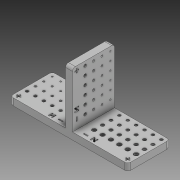
# Autodesk Inventor part: Drill Bushings Test Print
Saved by Autodesk Inventor 2022 (Build 260153000, 153)
## iProperties
Created: 2022-01-18
Part Number: Drill Bushings Test Print
Material: ABS Plastic
Document SubType Name: Modeling
Density: 1.06 g/cm^3
Appearance: Smooth - Medium Gray
Autodesk Inventor part; units mm, degrees
ref_plane "YZ Plane" through (0, 0, 0) normal (1, 0, 0) x (0, 1, 0)
ref_plane "XZ Plane" through (0, 0, 0) normal (0, 1, 0) x (-1, 0, 0)
ref_plane "XY Plane" through (0, 0, 0) normal (0, 0, 1) x (1, 0, 0)
sketch "Sketch1" plane through (0, 0, 0) normal (0, 1, 0) x (-1, 0, 0)
  line L0 (4.7625, 77.3906) -> (-4.7625, 77.3906)
  line L1 (-4.7625, 77.3906) -> (-4.7625, 75.0094)
  line L2 (-4.7625, 75.0094) -> (4.7625, 75.0094)
  line L3 (4.7625, 75.0094) -> (4.7625, 77.3906)
  line L4 (4.7625, 77.3906) -> (-4.7625, 75.0094) construction
  line L5 (-4.7625, 77.3906) -> (4.7625, 75.0094) construction
  line L6 (-90.4875, 77.3906) -> (-100.0125, 77.3906)
  line L7 (-100.0125, 77.3906) -> (-100.0125, 75.0094)
  line L8 (-100.0125, 75.0094) -> (-90.4875, 75.0094)
  line L9 (-90.4875, 75.0094) -> (-90.4875, 77.3906)
  line L10 (-90.4875, 77.3906) -> (-100.0125, 75.0094) construction
  line L11 (-100.0125, 77.3906) -> (-90.4875, 75.0094) construction
  line L12 (-96.4406, 71.4375) -> (-94.0594, 71.4375)
  line L13 (-94.0594, 71.4375) -> (-94.0594, 80.9625)
  line L14 (-94.0594, 80.9625) -> (-96.4406, 80.9625)
  line L15 (-96.4406, 80.9625) -> (-96.4406, 71.4375)
  line L16 (-96.4406, 71.4375) -> (-94.0594, 80.9625) construction
  line L17 (-94.0594, 71.4375) -> (-96.4406, 80.9625) construction
  line L18 (-14.2875, 80.9625) -> (-14.2875, 71.4375)
  line L19 (-14.2875, 71.4375) -> (-16.6687, 71.4375)
  line L20 (-16.6687, 71.4375) -> (-21.4312, 77.2177)
  line L21 (-21.4312, 77.2177) -> (-21.4312, 71.4375)
  line L22 (-21.4312, 71.4375) -> (-23.8125, 71.4375)
  line L23 (-23.8125, 71.4375) -> (-23.8125, 80.9625)
  line L24 (-23.8125, 80.9625) -> (-21.4312, 80.9625)
  line L25 (-21.4312, 80.9625) -> (-16.6687, 75.1823)
  line L26 (-16.6687, 75.1823) -> (-16.6687, 80.9625)
  line L27 (-16.6687, 80.9625) -> (-14.2875, 80.9625)
  line L28 (-19.05, 78.0724) -> (-19.05, 74.3276) construction
  line L29 (28.575, -9.525) -> (-104.775, -9.525)
  line L30 (-104.775, -9.525) -> (-104.775, 85.725)
  line L31 (-104.775, 85.725) -> (28.575, 85.725)
  line L32 (28.575, 85.725) -> (28.575, -9.525)
  line L33 (28.575, -9.525) -> (-104.775, 85.725) construction
  line L34 (-104.775, -9.525) -> (28.575, 85.725) construction
  point P0 (0, 76.2)
  point P1 (-95.25, 76.2)
  point P2 (-95.25, 76.2)
  point P3 (0, 76.2)
  point P4 (-95.25, 76.2)
  point P5 (0, 76.2)
  point P6 (-95.25, 76.2)
  point P7 (-96.4406, 77.3906)
  point P8 (-94.0594, 77.3906)
  point P9 (-94.0594, 75.0094)
  point P10 (-96.4406, 75.0094)
  point P11 (0, 0)
  point P12 (-19.05, 76.2)
  point P13 (-95.25, 76.2)
  point P14 (-19.05, 0)
  point P15 (-38.1, 0)
  point P16 (-57.15, 0)
  point P17 (-76.2, 0)
  point P18 (-38.1, 38.1)
  point P19 (-95.25, 0)
  point P20 (0, 19.05)
  point P21 (-19.05, 19.05)
  point P22 (-57.15, 19.05)
  point P23 (-38.1, 19.05)
  point P24 (-95.25, 19.05)
  point P25 (-76.2, 19.05)
  point P26 (0, 38.1)
  point P27 (-19.05, 38.1)
  point P28 (-57.15, 38.1)
  point P29 (-38.1, 38.1)
  point P30 (-95.25, 38.1)
  point P31 (-76.2, 38.1)
  point P32 (0, 57.15)
  point P33 (-19.05, 57.15)
  point P34 (-57.15, 57.15)
  point P35 (-38.1, 57.15)
  point P36 (-95.25, 57.15)
  point P37 (-76.2, 57.15)
  point P38 (28.575, 38.1)
  dimension "d137" = 25.4
  dimension "d33" = 9.525
  dimension "d34" = 2.3813
  dimension "d61" = 9.525
  dimension "d62" = 9.525
  dimension "d64" = 2.3813
  dimension "d67" = 133.35
  dimension "d81" = 19.05
  dimension "d123" = 0
  dimension "d134" = 19.05
  dimension "d139" = 19.05
  dimension "d140" = 9.525
  constraints: 71 end point, 17 midpoint, 11 parallel, 7 equal length, 7 perpendicular, 6 point on line, 5 horizontal, 4 vertical alignment, 3 horizontal alignment, 2 vertical, 23 other
  measures "d33" distance of L1.end L2.end
  measures "d34" distance of L2.end L0.start
  measures "d61" distance between parallel lines of L23 L18
  measures "d62" distance between parallel lines of L24 L22
  measures "d64" distance between parallel lines of L25 L20
  measures "d67" distance of L29.start L29.end
  measures "d81" distance of point (0, 0) point (-19.05, 0)
  measures "d123" horizontal distance of point (-38.1, 38.1) point (-38.1, 0)
  measures "d134" distance of point (0, 0) point (0, 19.05)
  measures "d139" distance of point (0, 76.2) point (0, 57.15)
  measures "d140" distance from line of point (0, 0) L29
extrude "Extrusion1" add sketch "Sketch1" against normal blind 15.875
fillet "Fillet1" radius 6.35 2 edges at (104.775, -7.9375, -9.525) (104.775, -7.9375, 85.725)
fillet "Fillet2" radius 0.3969 26 edges at (21.4312, -7.9375, 77.2177) (100.0125, -7.9375, 75.0094) (100.0125, -7.9375, 77.3906) (96.4406, -7.9375, 77.3906) (96.4406, -7.9375, 80.9625) (94.0594, -7.9375, 80.9625) (94.0594, -7.9375, 77.3906) (90.4875, -7.9375, 77.3906) (90.4875, -7.9375, 75.0094) (94.0594, -7.9375, 75.0094) (94.0594, -7.9375, 71.4375) (96.4406, -7.9375, 71.4375) (96.4406, -7.9375, 75.0094) (21.4312, -7.9375, 71.4375) (23.8125, -7.9375, 71.4375) (23.8125, -7.9375, 80.9625) (21.4312, -7.9375, 80.9625) (16.6687, -7.9375, 75.1823) (16.6687, -7.9375, 71.4375) (14.2875, -7.9375, 71.4375) (16.6687, -7.9375, 80.9625) (14.2875, -7.9375, 80.9625) (4.7625, -7.9375, 77.3906) (4.7625, -7.9375, 75.0094) (-4.7625, -7.9375, 75.0094) (-4.7625, -7.9375, 77.3906)
hole "Hole7" at (19.05, 0, 38.1) direction (0, -1, 0) diameter 6.35 depth 10.16 counterbore diameter 7.9375 counterbore depth 1.27 clearance for "Hex Head Bolt" size "1/4" standard "Ansi Unified Screw Threads"
hole "Hole8" at (0, 0, 38.1) direction (0, -1, 0) diameter 6.223 depth 10.16 counterbore diameter 7.8105 counterbore depth 1.27
hole "Hole9" at (38.1, 0, 38.1) direction (0, -1, 0) diameter 6.477 depth 10.16 counterbore diameter 8.0645 counterbore depth 1.27 clearance for "Hex Head Bolt" size "1/4" standard "Ansi Unified Screw Threads"
hole "Hole10" at (57.15, 0, 38.1) direction (0, -1, 0) diameter 6.604 depth 10.16 counterbore diameter 8.1915 counterbore depth 1.27 clearance for "Hex Head Bolt" size "1/4" standard "Ansi Unified Screw Threads"
hole "Hole11" at (76.2, 0, 38.1) direction (0, -1, 0) diameter 6.731 depth 10.16 counterbore diameter 8.3185 counterbore depth 1.27 clearance for "Hex Head Bolt" size "1/4" standard "Ansi Unified Screw Threads"
hole "Hole12" at (95.25, 0, 38.1) direction (0, -1, 0) diameter 6.858 depth 10.16 counterbore diameter 8.4455 counterbore depth 1.27 clearance for "Hex Head Bolt" size "1/4" standard "Ansi Unified Screw Threads"
hole "Hole13" at (19.05, 0, 0) direction (0, -1, 0) diameter 5.0546 depth 7.62 counterbore diameter 6.35 counterbore depth 1.016
hole "Hole14" at (0, 0, 0) direction (0, -1, 0) diameter 4.9276 depth 7.62 counterbore diameter 6.223 counterbore depth 1.016
hole "Hole15" at (38.1, 0, 0) direction (0, -1, 0) diameter 5.1816 depth 7.62 counterbore diameter 6.477 counterbore depth 1.016
hole "Hole16" at (76.2, 0, 0) direction (0, -1, 0) diameter 5.4356 depth 7.62 counterbore diameter 6.731 counterbore depth 1.016
hole "Hole17" at (57.15, 0, 0) direction (0, -1, 0) diameter 5.3086 depth 7.62 counterbore diameter 6.604 counterbore depth 1.016
hole "Hole18" at (95.25, 0, 0) direction (0, -1, 0) diameter 5.5626 depth 7.62 counterbore diameter 6.858 counterbore depth 1.016
hole "Hole19" at (19.05, 0, 57.15) direction (0, -1, 0) diameter 8.2804 depth 13.97 counterbore diameter 9.525 counterbore depth 1.524
hole "Hole20" at (0, 0, 57.15) direction (0, -1, 0) diameter 8.1534 depth 13.97 counterbore diameter 9.398 counterbore depth 1.524
hole "Hole21" at (38.1, 0, 57.15) direction (0, -1, 0) diameter 8.4074 depth 13.97 counterbore diameter 9.652 counterbore depth 1.524
hole "Hole22" at (57.15, 0, 57.15) direction (0, -1, 0) diameter 8.5344 depth 13.97 counterbore diameter 9.779 counterbore depth 1.524
hole "Hole23" at (76.2, 0, 57.15) direction (0, -1, 0) diameter 8.6614 depth 13.97 counterbore diameter 9.906 counterbore depth 1.524
hole "Hole24" at (95.25, 0, 57.15) direction (0, -1, 0) diameter 8.7884 depth 13.97 counterbore diameter 10.033 counterbore depth 1.524
hole "Hole25" at (19.05, 0, 19.05) direction (0, -1, 0) diameter 5.842 depth 8.89 counterbore diameter 7.112 counterbore depth 1.016
hole "Hole26" at (0, 0, 19.05) direction (0, -1, 0) diameter 5.715 depth 8.89 counterbore diameter 6.985 counterbore depth 1.016
hole "Hole27" at (38.1, 0, 19.05) direction (0, -1, 0) diameter 5.969 depth 8.89 counterbore diameter 7.239 counterbore depth 1.016
hole "Hole28" at (76.2, 0, 19.05) direction (0, -1, 0) diameter 6.223 depth 8.89 counterbore diameter 7.493 counterbore depth 1.016
hole "Hole29" at (57.15, 0, 19.05) direction (0, -1, 0) diameter 6.096 depth 8.89 counterbore diameter 7.366 counterbore depth 1.016
hole "Hole30" at (95.25, 0, 19.05) direction (0, -1, 0) diameter 6.35 depth 8.89 counterbore diameter 7.62 counterbore depth 1.016 clearance for "Hex Head Bolt" size "1/4" standard "Ansi Unified Screw Threads"
sketch "Sketch2" plane through (0, -7.62, 0) normal (0, 1, 0) x (1, 0, 0)
  circle A0 centre (0, 0) radius 2.4638 projected
  circle A1 centre (19.05, 0) radius 2.5273 projected
  circle A2 centre (38.1, 0) radius 2.5908 projected
  circle A3 centre (57.15, 0) radius 2.6543 projected
  circle A4 centre (76.2, 0) radius 2.7178 projected
  circle A5 centre (95.25, 0) radius 2.7813 projected
  constraints: 6 coincident
hole "Hole31" at (0, -7.62, 0) at (19.05, -7.62, 0) at (38.1, -7.62, 0) at (57.15, -7.62, 0) at (76.2, -7.62, 0) at (95.25, -7.62, 0) direction (0, -1, 0) diameter 3.556 end through all
sketch "Sketch3" plane through (0, -8.89, 19.05) normal (0, 1, 0) x (1, 0, 0)
  circle A0 centre (0, 0) radius 2.8575 projected
  circle A1 centre (19.05, 0) radius 2.921 projected
  circle A2 centre (38.1, 0) radius 2.9845 projected
  circle A3 centre (57.15, 0) radius 3.683 projected
  circle A4 centre (76.2, 0) radius 3.7465 projected
  circle A5 centre (95.25, 0) radius 3.81 projected
  point P0 (0, 19.05)
  constraints: 6 coincident
hole "Hole32" at (0, -8.89, 19.05) at (19.05, -8.89, 19.05) at (38.1, -8.89, 19.05) at (57.15, -8.89, 19.05) at (76.2, -8.89, 19.05) at (95.25, -8.89, 19.05) direction (0, -1, 0) diameter 4.318 end through all
sketch "Sketch4" plane through (0, -10.16, 38.1) normal (0, 1, 0) x (1, 0, 0)
  circle A0 centre (0, 0) radius 3.9052 projected
  circle A1 centre (19.05, 0) radius 3.9687 projected
  circle A2 centre (38.1, 0) radius 3.2385 projected
  circle A3 centre (57.15, 0) radius 3.302 projected
  circle A4 centre (76.2, 0) radius 3.3655 projected
  circle A5 centre (95.25, 0) radius 3.429 projected
  point P0 (0, 38.1)
  constraints: 6 coincident
hole "Hole33" at (0, -10.16, 38.1) at (19.05, -10.16, 38.1) at (38.1, -10.16, 38.1) at (57.15, -10.16, 38.1) at (76.2, -10.16, 38.1) at (95.25, -10.16, 38.1) direction (0, -1, 0) diameter 5.334 end through all
sketch "Sketch5" plane through (0, -13.97, 57.15) normal (0, 1, 0) x (1, 0, 0)
  circle A0 centre (0, 0) radius 4.699 projected
  circle A1 centre (19.05, 0) radius 4.7625 projected
  circle A2 centre (38.1, 0) radius 4.826 projected
  circle A3 centre (57.15, 0) radius 4.8895 projected
  circle A4 centre (76.2, 0) radius 4.953 projected
  circle A5 centre (95.25, 0) radius 5.0165 projected
  point P0 (0, 57.15)
  constraints: 6 coincident
hole "Hole34" at (0, -13.97, 57.15) at (19.05, -13.97, 57.15) at (38.1, -13.97, 57.15) at (57.15, -13.97, 57.15) at (76.2, -13.97, 57.15) at (95.25, -13.97, 57.15) direction (0, -1, 0) diameter 6.604 end through all
ref_plane "Work Plane1" through (0, -7.9375, 0) normal (0, 1, 0) x (1, 0, 0)
pattern_circular "Circular Pattern1" count 3 over 180 about axis through (-28.575, -7.9375, 0) along (0, 0, 1)
fillet "Fillet3" [suppressed]
body "Solid1"
